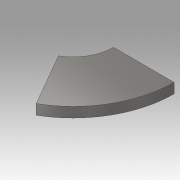
# Autodesk Inventor part: Arch 60
Saved by Autodesk Inventor 2019.1 (Build 231200000, 200)
## iProperties
Created: 2021-11-21
Part Number: Arch 60
Material: Сталь, мягкая
Description: =<Title>
Document SubType Name: Modeling
Density: 7.85 g/cm^3
Appearance: С умеренной полировкой
Autodesk Inventor part; units mm, degrees
ref_plane "YZ Plane" through (0, 0, 0) normal (1, 0, 0) x (0, 1, 0)
ref_plane "XZ Plane" through (0, 0, 0) normal (0, 1, 0) x (-1, 0, 0)
ref_plane "XY Plane" through (0, 0, 0) normal (0, 0, 1) x (1, 0, 0)
sketch "Эскиз2" plane through (0, 0, 0) normal (0, 1, 0) x (-1, 0, 0)
  line L0 (-1, 0) -> (-0.4, 0)
  arc A0 (-0.5, 0.866) -> (-1, 0) centre (0, 0) ccw
  line L1 (-0.2, 0.3464) -> (-0.5, 0.866) construction
  line L2 (0, 0) -> (-1, 0) construction
  line L3 (-0.5, 0.866) -> (-0.2, 0.3464)
  arc A1 (-0.2, 0.3464) -> (-0.4, 0) centre (0, 0) ccw
  dimension "d4" = 60
  dimension "d9" = 2
  dimension "d10" = 0.8
  constraints: 8 end point, 4 point on circle, 2 centre point, 2 coincident, 2 point on line, 1 collinear, 1 horizontal
  measures "d4" angle of L1 L2
  measures "d9" diameter of A0
  measures "d10" diameter of A1
extrude "Выдавливание2" add sketch "Эскиз2" along normal blind 0.1
